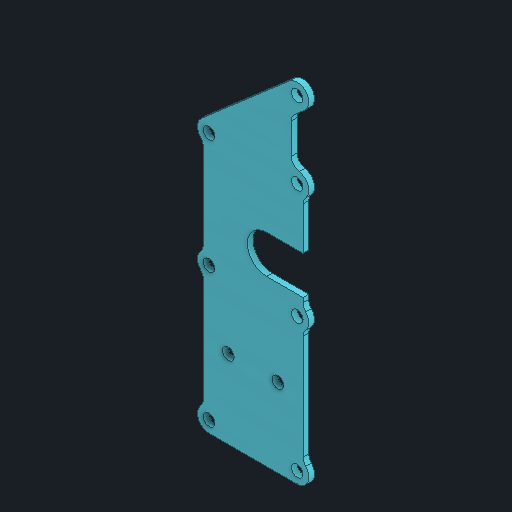
# Autodesk Inventor part: tibea_outside_steel
Saved by Autodesk Inventor 2026 (Build 300175000, 175)
## iProperties
Created: 2026-04-23
Part Number: tibea_outside_steel
Material: Сталь
Document SubType Name: Modeling
Designer: user
Density: 7.85 g/cm^3
Appearance: Серо-синий
Mass: 182.865 g
Surface Area: 175.758 cm^2
Volume: 23.2949 cm^3
Author: user
Autodesk Inventor part; units mm, degrees
ref_plane "YZ Plane" through (0, 0, 0) normal (1, 0, 0) x (0, 1, 0)
ref_plane "XZ Plane" through (0, 0, 0) normal (0, 1, 0) x (-1, 0, 0)
ref_plane "XY Plane" through (0, 0, 0) normal (0, 0, 1) x (1, 0, 0)
sketch "Эскиз1" plane through (0, 0, 0) normal (0, 0, 1) x (1, 0, 0)
  line L0 (-302.1837, 10.5492) -> (-302.1837, 99.2824)
  line L1 (-302.1837, 21.7824) -> (-325.2337, 21.7824)
  circle A0 centre (-325.2337, 27.8824) radius 3.05
  arc A1 (-329.6576, 32.0823) -> (-325.2337, 21.7824) centre (-325.2337, 27.8824) ccw
  circle A2 centre (-315.1337, 62.8824) radius 3.05
  line L2 (-328.2837, 35.5249) -> (-328.2837, 90.2399)
  arc A3 (-329.6576, 102.0823) -> (-329.6576, 93.6825) centre (-325.2337, 97.8824) ccw
  circle A4 centre (-325.2337, 97.8824) radius 3.05
  line L3 (-302.1837, 21.7824) -> (-279.1337, 21.7824)
  circle A5 centre (-279.1337, 27.8824) radius 3.05
  arc A6 (-279.1337, 21.7824) -> (-274.7099, 32.0823) centre (-279.1337, 27.8824) ccw
  circle A7 centre (-289.2337, 62.8824) radius 3.05
  line L4 (-276.0837, 35.5249) -> (-276.0837, 90.2399)
  arc A8 (-274.7099, 93.6825) -> (-274.7099, 102.0823) centre (-279.1337, 97.8824) ccw
  circle A9 centre (-279.1337, 97.8824) radius 3.05
  arc A10 (-295.1837, 127.8824) -> (-295.1837, 107.8824) centre (-295.1837, 117.8824) ccw
  line L5 (-328.2837, 105.5249) -> (-328.2837, 150.2399)
  arc A11 (-329.2315, 162.4898) -> (-329.6576, 153.6825) centre (-325.2337, 157.8824) ccw
  circle A12 centre (-325.2337, 157.8824) radius 3.05
  arc A13 (-274.7099, 153.6825) -> (-278.0621, 163.8875) centre (-279.1337, 157.8824) ccw
  circle A14 centre (-279.1337, 157.8824) radius 3.05
  circle A15 centre (-279.1337, 197.8824) radius 3.05
  arc A16 (-275.136, 193.275) -> (-283.1315, 202.4898) centre (-279.1337, 197.8824) ccw
  line L6 (-329.2315, 162.4898) -> (-283.1315, 202.4898)
  line L7 (-275.136, 193.275) -> (-280.4606, 188.655)
  line L8 (-295.1837, 107.8824) -> (-276.0837, 107.8824)
  line L9 (-295.1837, 127.8824) -> (-276.0837, 127.8824)
  line L10 (-276.0837, 105.5249) -> (-276.0837, 107.8824)
  line L11 (-276.0837, 127.8824) -> (-276.0837, 150.2399)
  line L12 (-282.1837, 168.8098) -> (-282.1837, 184.8784)
  arc A17 (-328.2837, 150.2399) -> (-329.6576, 153.6825) centre (-333.2837, 150.2399) ccw
  arc A18 (-328.2837, 90.2399) -> (-329.6576, 93.6825) centre (-333.2837, 90.2399) ccw
  arc A19 (-276.0837, 35.5249) -> (-274.7099, 32.0823) centre (-271.0837, 35.5249) ccw
  arc A20 (-329.6576, 32.0823) -> (-328.2837, 35.5249) centre (-333.2837, 35.5249) ccw
  arc A21 (-329.6576, 102.0823) -> (-328.2837, 105.5249) centre (-333.2837, 105.5249) ccw
  arc A22 (-274.7099, 93.6825) -> (-276.0837, 90.2399) centre (-271.0837, 90.2399) ccw
  arc A23 (-274.7099, 153.6825) -> (-276.0837, 150.2399) centre (-271.0837, 150.2399) ccw
  arc A24 (-276.0837, 105.5249) -> (-274.7099, 102.0823) centre (-271.0837, 105.5249) ccw
  arc A25 (-282.1837, 168.8098) -> (-278.0621, 163.8875) centre (-277.1837, 168.8098) ccw
  arc A26 (-280.4606, 188.655) -> (-282.1837, 184.8784) centre (-277.1837, 184.8784) ccw
  point P0 (-328.2837, 33.1651)
  point P1 (-328.2837, 92.5996)
  point P2 (-276.0837, 33.1651)
  point P3 (-276.0837, 92.5996)
  point P4 (-276.0837, 103.1651)
  point P5 (-276.0837, 152.5996)
  point P6 (-328.2837, 103.1651)
  point P7 (-282.1837, 203.1651)
  point P8 (-282.1837, 163.1651)
  point P9 (-328.2837, 152.5996)
  dimension "d0" = 6.1
  dimension "d1" = 12.2
  dimension "d2" = 46.1
  dimension "d10" = 70
  dimension "d11" = 35
  dimension "d12" = 10.1
  dimension "d13" = 20
  dimension "d15" = 55
  dimension "d17" = 7
  dimension "d18" = 40
  dimension "d19" = 40
  dimension "d20" = 5
  constraints: 46 point on circle, 28 tangent, 27 centre point, 26 end point, 18 equal radius, 10 point on line, 8 symmetric about line, 7 coincident, 6 vertical, 4 vertical alignment, 3 collinear, 2 horizontal, 2 perpendicular, 1 horizontal alignment, 1 parallel, 6 other
  measures "d0" diameter of A0
  measures "d1" diameter of A1
  measures "d2" diameter of A0.centre L0
  measures "d10" distance of A3.centre A0.centre
  measures "d11" vertical distance of A0.centre A2.centre
  measures "d12" horizontal distance of A2.centre A0.centre
  measures "d13" diameter of A10
  measures "d15" vertical distance of A10.centre A7.centre
  measures "d17" distance from line of L0 A10.centre
  measures "d18" vertical distance of A10.centre A11.centre
  measures "d19" distance of A16.centre A13.centre
  measures "d20" radius of A17
extrude "Выдавливание1" add sketch "Эскиз1" along normal blind 3
equation "\"d0\" = d_main_screw_holes"
equation "\"d1\" = 2 * d_main_screw_holes"
equation "\"d2\" = hight_profile_tibea + d_main_screw_holes"
equation "\"d12\" = d_main_screw_holes + thickness_profile_tibea"
equation "\"d13\" = d_main_shaft"
equation "\"d21\" = thickness_steel"
equation "\"tolerance_plazma\" = 0.1"
equation "\"thickness_steel\" = 3"
equation "\"d_main_screw_holes\" = 6.1"
equation "\"d_main_shaft\" = 20"
equation "\"thickness_profile_tibea\" = 4"
equation "\"hight_profile_tibea\" = 40"
equation "\"thickness_profile_femur\" = 3"
equation "\"width_shaft_shift\" = 35"
equation "\"width_flattened_surface\" = 12"
